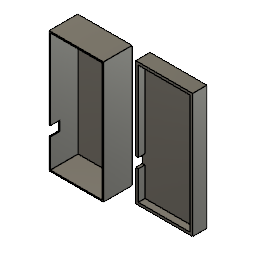
NES Case v6 (Autodesk Fusion 360 design; units mm, degrees)
Autodesk Fusion 360 part; units mm, degrees
sketch "Sketch1" plane through (0, 0, 0) normal (0, 0, 1) x (1, 0, 0)
  line L0 (0, 0) -> (54, 0)
  line L1 (54, 0) -> (54, 124)
  line L2 (54, 124) -> (0, 124)
  line L3 (0, 124) -> (0, 0)
  line L4 (54, 0) -> (55.4142, -1.4142)
  line L5 (54, 0) -> (56, 0) construction
  line L6 (0, 124) -> (-1.4142, 125.4142)
  line L7 (-1.4142, 125.4142) -> (55.4142, 125.4142)
  line L8 (55.4142, 125.4142) -> (55.4142, -1.4142)
  line L9 (55.4142, -1.4142) -> (-1.4142, -1.4142)
  line L10 (-1.4142, -1.4142) -> (-1.4142, 125.4142)
  dimension "d1" = 54
  dimension "d2" = 124
  dimension "d3" = 2
  dimension "d4" = 45
  dimension "d5" = 2
  constraint horizontal L0
  constraint vertical L1
  constraint horizontal L2
  constraint vertical L3
  constraint coincident L0.start L3.end
  constraint horizontal L5
  constraint horizontal L7
  constraint vertical L8
  constraint horizontal L9
  constraint vertical L10
  measures "d1" distance of L0.start L0.end
  measures "d2" distance of L0.start L2.end
  measures "d3" distance of L0.end L4.end
  measures "d4" angle of L4 L5
  measures "d5" distance of L2.end L6.end
extrude "Extrude1" add sketch "Sketch1" along normal blind 30 contours L0 L3 L4 L6 L9 L10 | L1 L2 L4 L6 L7 L8 makes body 1
sketch "Sketch2" plane through (0, 0, 0) normal (0, 0, 1) x (1, 0, 0)
  line L0 (-1.4142, -1.4142) -> (55.4142, -1.4142)
  line L1 (55.4142, -1.4142) -> (55.4142, 125.4142)
  line L2 (55.4142, 125.4142) -> (-1.4142, 125.4142)
  line L3 (-1.4142, 125.4142) -> (-1.4142, -1.4142)
  point P0 (-1.4142, -1.4142)
  point P1 (55.4142, 125.4142)
  constraint horizontal L0
  constraint vertical L1
  constraint horizontal L2
  constraint vertical L3
  constraint coincident P1 L1.end
  constraint coincident P0 L0.start
extrude "Extrude2" add sketch "Sketch2" along normal blind 1 bodies 1
sketch "Sketch3" plane through (0, 0, 0) normal (0, 0, 1) x (1, 0, 0)
  line L0 (70, 0) -> (128, 0)
  line L1 (128, 0) -> (128, 128)
  line L2 (128, 128) -> (70, 128)
  line L3 (70, 128) -> (70, 0)
  line L4 (70, 0) -> (70.7071, 0.7071)
  line L5 (128, 128) -> (127.2929, 127.2929)
  line L6 (127.2929, 127.2929) -> (70.7071, 127.2929)
  line L7 (70.7071, 127.2929) -> (70.7071, 0.7071)
  line L8 (70.7071, 0.7071) -> (127.2929, 0.7071)
  line L9 (127.2929, 0.7071) -> (127.2929, 127.2929)
  dimension "d10" = 58
  dimension "d11" = 128
  dimension "d12" = 1
  dimension "d13" = 1
  constraint horizontal L0
  constraint vertical L1
  constraint horizontal L2
  constraint vertical L3
  constraint horizontal L6
  constraint vertical L7
  constraint horizontal L8
  constraint vertical L9
  measures "d10" distance of L0.start L0.end
  measures "d11" distance of L0.start L2.end
  measures "d12" distance of L0.start L4.end
  measures "d13" distance of L1.end L5.end
sketch "Sketch8" plane through (0, 0, 30) normal (0, 0, 1) x (1, 0, 0)
  line L0 (0, 0) -> (0, 124)
  line L1 (0, 124) -> (54, 124)
  line L2 (54, 124) -> (54, 0)
  line L3 (54, 0) -> (0, 0)
  line L4 (-1.4142, -1.4142) -> (55.4142, -1.4142)
  line L5 (55.4142, -1.4142) -> (55.4142, 125.4142)
  line L6 (55.4142, 125.4142) -> (-1.4142, 125.4142)
  line L7 (-1.4142, 125.4142) -> (-1.4142, -1.4142)
  line L8 (-1.4142, -1.4142) -> (-1.4142, 29.9998)
  line L9 (-1.4142, 29.9998) -> (0, 29.9998)
  line L10 (0, 29.9998) -> (0, 39.9998)
  line L11 (0, 39.9998) -> (-1.4142, 39.9998)
  line L12 (-1.4142, 39.9998) -> (-1.4142, 29.9998)
  dimension "d30" = 31.414
  dimension "d31" = 10
  constraint coincident L4.start L7.end
  constraint horizontal L9
  constraint vertical L10
  constraint horizontal L11
  constraint vertical L12
  measures "d30" distance of L4.start L8.end
  measures "d31" distance of L8.end L11.end
extrude "Extrude9" cut sketch "Sketch8" against normal blind 10 contours L0 L7 L9 L10 L11 L12 bodies 1
sketch "Sketch9" plane through (0, 0, 0) normal (0, 0, 1) x (1, 0, 0)
  line L0 (75, 0) -> (132.5, 0)
  line L1 (132.5, 0) -> (132.5, 127.5)
  line L2 (132.5, 127.5) -> (75, 127.5)
  line L3 (75, 127.5) -> (75, 0)
  line L4 (75, 127.5) -> (74.2929, 128.2071)
  line L5 (75, 127.5) -> (76, 127.5) construction
  line L6 (132.5, 0) -> (133.2071, -0.7071)
  line L7 (132.5, 0) -> (133.5, 0) construction
  line L8 (133.2071, -0.7071) -> (74.2929, -0.7071)
  line L9 (74.2929, -0.7071) -> (74.2929, 128.2071)
  line L10 (74.2929, 128.2071) -> (133.2071, 128.2071)
  line L11 (133.2071, 128.2071) -> (133.2071, -0.7071)
  dimension "d40" = 57.5
  dimension "d41" = 127.5
  dimension "d42" = 135
  dimension "d43" = 1
  dimension "d44" = 45
  dimension "d45" = 1
  constraint horizontal L0
  constraint vertical L1
  constraint horizontal L2
  constraint vertical L3
  constraint horizontal L5
  constraint horizontal L7
  constraint horizontal L8
  constraint vertical L9
  constraint horizontal L10
  constraint vertical L11
  measures "d40" distance of L0.start L0.end
  measures "d41" distance of L0.start L2.end
  measures "d42" angle of L4 L5
  measures "d43" distance of L2.end L4.end
  measures "d44" angle of L6 L7
  measures "d45" distance of L0.end L6.end
extrude "Extrude13" add sketch "Sketch9" along normal blind 7 separate body contours L0 L3 L4 L6 L8 L9 | L1 L2 L4 L6 L10 L11 makes body 2
sketch "Sketch10" plane through (0, 0, 7) normal (0, 0, 1) x (1, 0, 0)
  line L0 (75, 0) -> (75, 127.5)
  line L1 (75, 127.5) -> (132.5, 127.5)
  line L2 (132.5, 127.5) -> (132.5, 0)
  line L3 (132.5, 0) -> (75, 0)
  line L4 (133.2071, 128.2071) -> (74.2929, 128.2071)
  line L5 (74.2929, 128.2071) -> (74.2929, -0.7071)
  line L6 (74.2929, -0.7071) -> (133.2071, -0.7071)
  line L7 (133.2071, -0.7071) -> (133.2071, 128.2071)
extrude "Extrude14" add sketch "Sketch10" along normal blind 1 contours L0 L1 L2 L3 | L4 L5 L6 L7 bodies 2
sketch "Sketch11" plane through (0, 0, 8) normal (0, 0, 1) x (1, 0, 0)
  line L0 (133.2071, -0.7071) -> (133.2071, 128.2071)
  line L1 (133.2071, 128.2071) -> (74.2929, 128.2071)
  line L2 (74.2929, 128.2071) -> (74.2929, -0.7071)
  line L3 (74.2929, -0.7071) -> (133.2071, -0.7071)
  line L4 (133.2071, -0.7071) -> (131.0858, 1.4142)
  line L5 (133.2071, -0.7071) -> (136.2071, -0.7071) construction
  line L6 (74.2929, 128.2071) -> (76.4142, 126.0858)
  line L7 (74.2929, 128.2071) -> (77.2929, 128.2071) construction
  line L8 (76.4142, 126.0858) -> (131.0858, 126.0858)
  line L9 (131.0858, 126.0858) -> (131.0858, 1.4142)
  line L10 (131.0858, 1.4142) -> (76.4142, 1.4142)
  line L11 (76.4142, 1.4142) -> (76.4142, 126.0858)
  dimension "d50" = 135
  dimension "d51" = 3
  dimension "d52" = 45
  dimension "d53" = 3
  constraint coincident L0.start L3.end
  constraint horizontal L5
  constraint coincident L1.end L2.start
  constraint horizontal L7
  constraint horizontal L8
  constraint vertical L9
  constraint horizontal L10
  constraint vertical L11
  measures "d50" angle of L4 L5
  measures "d51" distance of L0.start L4.end
  measures "d52" angle of L6 L7
  measures "d53" distance of L1.end L6.end
extrude "Extrude15" add sketch "Sketch11" along normal blind 4 contours L0 L1 L4 L6 L8 L9 | L2 L3 L4 L6 L10 L11 bodies 2
sketch "Sketch12" plane through (0, 0, 12) normal (0, 0, 1) x (1, 0, 0)
  line L0 (131.0858, 1.4142) -> (76.4142, 1.4142)
  line L1 (76.4142, 1.4142) -> (76.4142, 126.0858)
  line L2 (76.4142, 126.0858) -> (131.0858, 126.0858)
  line L3 (131.0858, 126.0858) -> (131.0858, 1.4142)
  line L4 (74.2929, -0.7071) -> (133.2071, -0.7071)
  line L5 (133.2071, -0.7071) -> (133.2071, 128.2071)
  line L6 (133.2071, 128.2071) -> (74.2929, 128.2071)
  line L7 (74.2929, 128.2071) -> (74.2929, -0.7071)
  line L8 (76.4142, 1.4142) -> (76.4142, 32.0412)
  line L9 (76.4142, 32.0412) -> (74.2929, 32.0412)
  line L10 (74.2929, 32.0412) -> (74.2929, 42.0412)
  line L11 (74.2929, 42.0412) -> (76.4142, 42.0412)
  line L12 (76.4142, 42.0412) -> (76.4142, 32.0412)
  dimension "d56" = 30.627
  dimension "d57" = 10
  constraint coincident L0.end L1.start
  constraint horizontal L9
  constraint vertical L10
  constraint horizontal L11
  constraint vertical L12
  measures "d56" distance of L0.end L8.end
  measures "d57" distance of L8.end L11.end
extrude "Extrude16" cut sketch "Sketch12" against normal blind 32 contours L1 L7 L9 L10 L11 L12 bodies 2
extrude "Extrude17" add 1 faces at (76.4142, 35.3745, 7.6667) along direction (-1, 0, 0) blind 2.121 on bodies 2 bodies 2
extrude "Extrude18" add 1 faces at (74.2929, 70.7632, 8) along direction (-1, 0, 0) blind 0.3 on bodies 2 bodies 2
extrude "Extrude19" cut 1 faces at (73.9929, 70.7632, 8) along direction (1, 0, 0) blind 0.007 on bodies 2 bodies 2
extrude "Extrude20" add 1 faces at (74.2929, 21.1251, 4) along direction (-1, 0, 0) blind 0.297 on bodies 2 bodies 2
extrude "Extrude21" cut 1 faces at (73.9959, 21.1251, 4) along direction (1, 0, 0) blind 0.004 on bodies 2 bodies 2
extrude "Extrude22" add 1 faces at (74.2932, 35.3745, 7.6667) along direction (-1, 0, 0) blind 0.3 on bodies 2 bodies 2
extrude "Extrude23" add 1 faces at (133.2071, 85.2357, 8) along direction (1, 0, 0) blind 0.3 on bodies 2 bodies 2
extrude "Extrude24" cut 1 faces at (133.5071, 85.2357, 8) along direction (-1, 0, 0) blind 0.007 on bodies 2 bodies 2
extrude "Extrude25" add 1 faces at (93.8333, 128.2071, 4) along direction (0, 1, 0) blind 0.3 on bodies 2 bodies 2
extrude "Extrude26" cut 1 faces at (93.8333, 128.5071, 4) along direction (0, -1, 0) blind 0.007 on bodies 2 bodies 2
extrude "Extrude27" add 1 faces at (113.6667, -0.7071, 4) along direction (0, -1, 0) blind 0.3 on bodies 2 bodies 2
extrude "Extrude28" cut 1 faces at (113.6667, -1.0071, 4) along direction (0, 1, 0) blind 0.007 on bodies 2 bodies 2
extrude "Extrude29" add 2 faces at (76.4142, 70.0561, 9.3333) (76.4142, 21.8322, 10.6667) along direction (1, 0, 0) blind 0.336 on bodies 2 bodies 2
extrude "Extrude30" add 1 faces at (131.0858, 84.5286, 9.3333) along direction (-1, 0, 0) blind 0.336 on bodies 2 bodies 2
extrude "Extrude31" add 1 faces at (94.7501, 126.0858, 10.6667) along direction (0, -1, 0) blind 0.336 on bodies 2 bodies 2
extrude "Extrude32" add 1 faces at (112.7499, 1.4142, 9.3333) along direction (0, 1, 0) blind 0.336 on bodies 2 bodies 2
extrude "Extrude33" add 1 faces at (132.5833, 43.0834, 12) along direction (0, 0, 1) blind 3 on bodies 2 bodies 2
